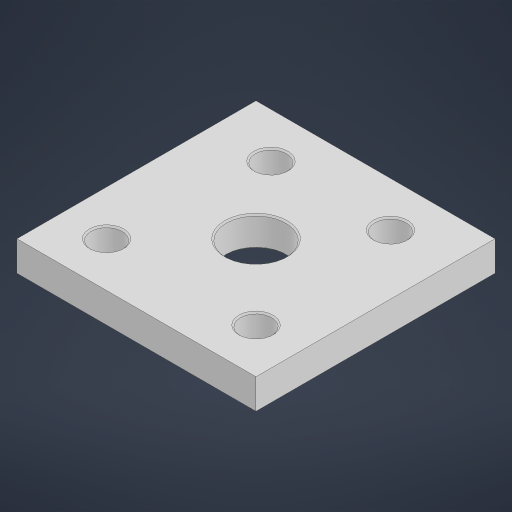
# Autodesk Inventor part: AP1-002
Saved by Autodesk Inventor 2024.3 (Build 283343000, 343)
## iProperties
Created: 2024-05-02
Part Number: AP1-002
Material: Generic
Document SubType Name: Modeling
Designer: fablabadmin
Density: 1 g/cm^3
Appearance: Default
Description: Plate top
Author: fablabadmin
Autodesk Inventor part; units mm, degrees
ref_plane "YZ Plane" through (0, 0, 0) normal (1, 0, 0) x (0, 1, 0)
ref_plane "XZ Plane" through (0, 0, 0) normal (0, 1, 0) x (-1, 0, 0)
ref_plane "XY Plane" through (0, 0, 0) normal (0, 0, 1) x (1, 0, 0)
sketch "Sketch1" plane through (0, 0, 0) normal (0, 1, 0) x (-1, 0, 0)
  line L0 (-40, 40) -> (40, 40)
  line L1 (40, 40) -> (40, -40)
  line L2 (40, -40) -> (-40, -40)
  line L3 (-40, -40) -> (-40, 40)
  line L4 (-40, 40) -> (40, -40) construction
  line L5 (40, 40) -> (-40, -40) construction
  line L6 (-25, 25) -> (25, 25) construction
  line L7 (25, 25) -> (25, -25) construction
  line L8 (25, -25) -> (-25, -25) construction
  line L9 (-25, -25) -> (-25, 25) construction
  line L10 (-25, 25) -> (25, -25) construction
  line L11 (25, 25) -> (-25, -25) construction
  line L12 (-20, 25) -> (20, 25) construction
  line L13 (20, 25) -> (20, -25) construction
  line L14 (20, -25) -> (-20, -25) construction
  line L15 (-20, -25) -> (-20, 25) construction
  line L16 (-20, 25) -> (20, -25) construction
  line L17 (20, 25) -> (-20, -25) construction
  circle A0 centre (0, 0) radius 10
  dimension "d0" = 80
  dimension "d1" = 50
  dimension "d2" = 40
  dimension "d3" = 20
  constraints: 36 end point, 6 midpoint, 6 parallel, 5 coincident, 5 perpendicular, 3 horizontal, 1 centre point, 1 point on line
  measures "d0" distance of L1.end L2.end
  measures "d1" distance of L7.end L8.end
  measures "d2" distance between parallel lines of L15 L13
  measures "d3" diameter of A0
extrude "Extrusion1" add sketch "Sketch1" against normal blind 10
hole "Hole1" at (-20, 0, -25) at (20, 0, -25) at (-25, 0, 25) at (25, 0, 25) direction (0, -1, 0) diameter 10.5 end through all
chamfer "Chamfer1" distance 0.5 angle 45 10 edges at (20, 0, -30.25) (-20, 0, -30.25) (25, 0, 19.75) (-25, 0, 19.75) (20, -10, -30.25) (-20, -10, -30.25) (25, -10, 19.75) (-25, -10, 19.75) (10, 0, 0) (10, -10, 0)
body "Solid1"
